Autodesk Fusion 360 part; units mm, degrees
note: some values were not read from the file. Set by a fixed rule: which sketch regions a step uses.
(part 6 of 20)
  spline S30 degree 5 poles (5.1346, -28.5878) (5.1347, -28.5879) (5.1347, -28.5881) (5.1348, -28.5884) (5.1349, -28.5889) (5.135, -28.5896) (5.1352, -28.5905) (5.1354, -28.5915) (5.1356, -28.5925) (5.1358, -28.5937) (5.1361, -28.595) (5.1363, -28.5964) (5.1367, -28.5979) (5.137, -28.5995) (5.1374, -28.6012) (5.1377, -28.603) (5.1381, -28.6049) (5.1386, -28.6069) (5.139, -28.6089) (5.1395, -28.6111) (5.14, -28.6134) (5.1406, -28.6158) (5.1411, -28.6182) (5.1417, -28.6208) (5.1423, -28.6234) (5.143, -28.6262) (5.1436, -28.629) (5.1443, -28.6319) (5.145, -28.6349) (5.1458, -28.6379) (5.1465, -28.6411) (5.1473, -28.6443) (5.1481, -28.6477) (5.149, -28.6511) (5.1499, -28.6545) (5.1508, -28.6581) (5.1517, -28.6617) (5.1527, -28.6655) (5.1536, -28.6693) (5.1546, -28.6731) (5.1557, -28.6771) (5.1567, -28.6811) (5.1578, -28.6852) (5.1589, -28.6893) (5.1601, -28.6936) (5.1613, -28.6979) (5.1625, -28.7023) (5.1637, -28.7067) (5.1649, -28.7112) (5.1662, -28.7158) (5.1675, -28.7205) (5.1689, -28.7252) (5.1702, -28.73) (5.1716, -28.7349) (5.173, -28.7398) (5.1745, -28.7448) (5.176, -28.7498) (5.1775, -28.7549) (5.179, -28.7601) (5.1806, -28.7654) (5.1822, -28.7707) (5.1838, -28.776) (5.1854, -28.7815) (5.1871, -28.7869) (5.1888, -28.7925) (5.1905, -28.7981) (5.1923, -28.8038) (5.1941, -28.8095) (5.1959, -28.8153) (5.1978, -28.8211) (5.1996, -28.827) (5.2015, -28.833) (5.2035, -28.839) (5.2054, -28.8451) (5.2074, -28.8512) (5.2094, -28.8573) (5.2115, -28.8636) (5.2136, -28.8699) (5.2157, -28.8762) (5.2178, -28.8826) (5.22, -28.889) (5.2222, -28.8955) (5.2244, -28.9021) (5.2266, -28.9087) (5.2289, -28.9153) (5.2312, -28.922) (5.2336, -28.9288) (5.2359, -28.9356) (5.2383, -28.9424) (5.2408, -28.9493) (5.2432, -28.9563) (5.2457, -28.9633) (5.2482, -28.9703) (5.2508, -28.9774) (5.2533, -28.9846) (5.2559, -28.9918) (5.2586, -28.999) (5.2612, -29.0063) (5.2639, -29.0136) (5.2666, -29.021) (5.2694, -29.0284) (5.2722, -29.0358) (5.275, -29.0433) (5.2778, -29.0509) (5.2807, -29.0585) (5.2836, -29.0661) (5.2865, -29.0738) (5.2895, -29.0815) (5.2925, -29.0893) (5.2955, -29.0971) (5.2986, -29.105) (5.3016, -29.1129) (5.3047, -29.1208) (5.3079, -29.1288) (5.3111, -29.1368) (5.3143, -29.1448) (5.3175, -29.1529) (5.3207, -29.1611) (5.324, -29.1692) (5.3273, -29.1775) (5.3307, -29.1857) (5.3341, -29.194) (5.3375, -29.2023) (5.3409, -29.2107) (5.3444, -29.2191) (5.3479, -29.2276) (5.3514, -29.2361) (5.355, -29.2446) (5.3586, -29.2531) (5.3622, -29.2617) (5.3658, -29.2704) (5.3695, -29.279) (5.3732, -29.2878) (5.377, -29.2965) (5.3807, -29.3053) (5.3846, -29.3141) (5.3884, -29.3229) (5.3922, -29.3318) (5.3961, -29.3407) (5.4001, -29.3497) (5.404, -29.3587) (5.408, -29.3677) (5.412, -29.3767) (5.4161, -29.3858) (5.4201, -29.395) (5.4242, -29.4041) (5.4284, -29.4133) (5.4325, -29.4225) (5.4367, -29.4318) (5.441, -29.441) (5.4452, -29.4504) (5.4495, -29.4597) (5.4538, -29.4691) (5.4582, -29.4785) (5.4625, -29.4879) (5.467, -29.4974) (5.4714, -29.5069) (5.4759, -29.5165) (5.4804, -29.526) (5.4849, -29.5356) (5.4895, -29.5452) (5.494, -29.5549) (5.4987, -29.5646) (5.5033, -29.5743) (5.508, -29.584) (5.5127, -29.5938) (5.5175, -29.6036) (5.5222, -29.6134) (5.527, -29.6233) (5.5319, -29.6332) (5.5367, -29.6431) (5.5416, -29.653) (5.5466, -29.663) (5.5515, -29.673) (5.5565, -29.683) (5.5615, -29.6931) (5.5666, -29.7032) (5.5717, -29.7133) (5.5768, -29.7234) (5.5819, -29.7336) (5.5871, -29.7437) (5.5923, -29.754) (5.5975, -29.7642) (5.6028, -29.7745) (5.6081, -29.7847) (5.6134, -29.7951) (5.6188, -29.8054) (5.6242, -29.8158) (5.6296, -29.8262) (5.635, -29.8366) (5.6405, -29.847) (5.646, -29.8575) (5.6515, -29.868) (5.6571, -29.8785) (5.6627, -29.889) (5.6683, -29.8996) (5.674, -29.9102) (5.6797, -29.9208) (5.6854, -29.9314) (5.6912, -29.9421) (5.697, -29.9527) (5.7028, -29.9634) (5.7086, -29.9742) (5.7145, -29.9849) (5.7204, -29.9957) (5.7263, -30.0065) (5.7323, -30.0173) (5.7383, -30.0281) (5.7443, -30.039) (5.7504, -30.0499) (5.7565, -30.0608) (5.7626, -30.0717) (5.7688, -30.0826) (5.7749, -30.0936) (5.7811, -30.1046) (5.7874, -30.1156) (5.7937, -30.1266) (5.8, -30.1377) (5.8063, -30.1487) (5.8127, -30.1598) (5.8191, -30.1709) (5.8255, -30.1821) (5.8319, -30.1932) (5.8384, -30.2044) (5.8449, -30.2156) (5.8515, -30.2268) (5.8581, -30.238) (5.8647, -30.2492) (5.8713, -30.2605) (5.878, -30.2718) (5.8847, -30.2831) (5.8914, -30.2944) (5.8982, -30.3058) (5.905, -30.3171) (5.9118, -30.3285) (5.9187, -30.3399) (5.9255, -30.3513) (5.9325, -30.3628) (5.9394, -30.3742) (5.9464, -30.3857) (5.9534, -30.3972) (5.959, -30.4064) (5.9633, -30.4133) (5.9661, -30.4179) (5.9675, -30.4202) knots 0 0 0 0 0 0 0.00416667 0.00833333 0.0125 0.01666667 0.02083333 0.025 0.02916667 0.03333333 0.0375 0.04166667 0.04583333 0.05 0.05416667 0.05833333 0.0625 0.06666667 0.07083333 0.075 0.07916667 0.08333333 0.0875 0.09166667 0.09583333 0.1 0.10416667 0.10833333 0.1125 0.11666667 0.12083333 0.125 0.12916667 0.13333333 0.1375 0.14166667 0.14583333 0.15 0.15416667 0.15833333 0.1625 0.16666667 0.17083333 0.175 0.17916667 0.18333333 0.1875 0.19166667 0.19583333 0.2 0.20416667 0.20833333 0.2125 0.21666667 0.22083333 0.225 0.22916667 0.23333333 0.2375 0.24166667 0.24583333 0.25 0.25416667 0.25833333 0.2625 0.26666667 0.27083333 0.275 0.27916667 0.28333333 0.2875 0.29166667 0.29583333 0.3 0.30416667 0.30833333 0.3125 0.31666667 0.32083333 0.325 0.32916667 0.33333333 0.3375 0.34166667 0.34583333 0.35 0.35416667 0.35833333 0.3625 0.36666667 0.37083333 0.375 0.37916667 0.38333333 0.3875 0.39166667 0.39583333 0.4 0.40416667 0.40833333 0.4125 0.41666667 0.42083333 0.425 0.42916667 0.43333333 0.4375 0.44166667 0.44583333 0.45 0.45416667 0.45833333 0.4625 0.46666667 0.47083333 0.475 0.47916667 0.48333333 0.4875 0.49166667 0.49583333 0.5 0.50416667 0.50833333 0.5125 0.51666667 0.52083333 0.525 0.52916667 0.53333333 0.5375 0.54166667 0.54583333 0.55 0.55416667 0.55833333 0.5625 0.56666667 0.57083333 0.575 0.57916667 0.58333333 0.5875 0.59166667 0.59583333 0.6 0.60416667 0.60833333 0.6125 0.61666667 0.62083333 0.625 0.62916667 0.63333333 0.6375 0.64166667 0.64583333 0.65 0.65416667 0.65833333 0.6625 0.66666667 0.67083333 0.675 0.67916667 0.68333333 0.6875 0.69166667 0.69583333 0.7 0.70416667 0.70833333 0.7125 0.71666667 0.72083333 0.725 0.72916667 0.73333333 0.7375 0.74166667 0.74583333 0.75 0.75416667 0.75833333 0.7625 0.76666667 0.77083333 0.775 0.77916667 0.78333333 0.7875 0.79166667 0.79583333 0.8 0.80416667 0.80833333 0.8125 0.81666667 0.82083333 0.825 0.82916667 0.83333333 0.8375 0.84166667 0.84583333 0.85 0.85416667 0.85833333 0.8625 0.86666667 0.87083333 0.875 0.87916667 0.88333333 0.8875 0.89166667 0.89583333 0.9 0.90416667 0.90833333 0.9125 0.91666667 0.92083333 0.925 0.92916667 0.93333333 0.9375 0.94166667 0.94583333 0.95 0.95416667 0.95833333 0.9625 0.96666667 0.97083333 0.975 0.97916667 0.98333333 0.9875 0.99166667 0.99583333 1 1 1 1 1 1
  line L63 (2.1182, -28.9671) -> (2.1183, -28.9679)
  arc A27 (6.8665, -27.918) -> (8.0125, -27.6109) centre (0, 0) ccw
  arc A28 (5.9675, -30.4202) -> (6.9214, -30.2174) centre (0, 0) ccw
  line L64 (0.9213, -29.0298) -> (0.9119, -28.7355)
  line L65 (0.9213, -29.0307) -> (0.9213, -29.0298)
  line L66 (29.0307, 0.9213) -> (29.0298, 0.9213)
  spline S31 degree 5 poles (8.0948, -27.8945) (8.0948, -27.8946) (8.0948, -27.8948) (8.0949, -27.8951) (8.0951, -27.8956) (8.0953, -27.8963) (8.0956, -27.8971) (8.0958, -27.898) (8.0962, -27.8991) (8.0965, -27.9002) (8.0969, -27.9015) (8.0973, -27.9028) (8.0978, -27.9043) (8.0983, -27.9058) (8.0988, -27.9075) (8.0994, -27.9092) (8.1, -27.9111) (8.1007, -27.913) (8.1013, -27.915) (8.102, -27.9172) (8.1028, -27.9194) (8.1036, -27.9217) (8.1044, -27.9241) (8.1052, -27.9265) (8.1061, -27.9291) (8.107, -27.9318) (8.108, -27.9345) (8.109, -27.9373) (8.11, -27.9402) (8.1111, -27.9432) (8.1121, -27.9462) (8.1133, -27.9494) (8.1144, -27.9526) (8.1156, -27.9559) (8.1169, -27.9593) (8.1181, -27.9627) (8.1194, -27.9662) (8.1208, -27.9698) (8.1222, -27.9735) (8.1236, -27.9772) (8.125, -27.9811) (8.1265, -27.9849) (8.128, -27.9889) (8.1295, -27.9929) (8.1311, -27.997) (8.1327, -28.0012) (8.1344, -28.0054) (8.1361, -28.0097) (8.1378, -28.0141) (8.1395, -28.0185) (8.1413, -28.023) (8.1432, -28.0276) (8.145, -28.0322) (8.1469, -28.0369) (8.1488, -28.0416) (8.1508, -28.0464) (8.1528, -28.0513) (8.1548, -28.0562) (8.1569, -28.0612) (8.159, -28.0663) (8.1611, -28.0714) (8.1633, -28.0765) (8.1655, -28.0818) (8.1677, -28.087) (8.17, -28.0924) (8.1723, -28.0978) (8.1747, -28.1032) (8.177, -28.1087) (8.1795, -28.1143) (8.1819, -28.1199) (8.1844, -28.1256) (8.1869, -28.1313) (8.1895, -28.1371) (8.192, -28.1429) (8.1947, -28.1488) (8.1973, -28.1547) (8.2, -28.1607) (8.2027, -28.1667) (8.2055, -28.1728) (8.2083, -28.179) (8.2111, -28.1851) (8.214, -28.1914) (8.2169, -28.1977) (8.2198, -28.204) (8.2227, -28.2104) (8.2257, -28.2168) (8.2288, -28.2233) (8.2318, -28.2298) (8.2349, -28.2363) (8.2381, -28.2429) (8.2412, -28.2496) (8.2445, -28.2563) (8.2477, -28.263) (8.251, -28.2698) (8.2543, -28.2767) (8.2576, -28.2835) (8.261, -28.2905) (8.2644, -28.2974) (8.2678, -28.3044) (8.2713, -28.3115) (8.2748, -28.3186) (8.2784, -28.3257) (8.282, -28.3329) (8.2856, -28.3401) (8.2892, -28.3473) (8.2929, -28.3546) (8.2966, -28.3619) (8.3004, -28.3693) (8.3042, -28.3767) (8.308, -28.3842) (8.3118, -28.3917) (8.3157, -28.3992) (8.3196, -28.4068) (8.3236, -28.4144) (8.3276, -28.422) (8.3316, -28.4297) (8.3357, -28.4374) (8.3398, -28.4452) (8.3439, -28.4529) (8.348, -28.4608) (8.3522, -28.4686) (8.3565, -28.4765) (8.3607, -28.4845) (8.365, -28.4924) (8.3693, -28.5004) (8.3737, -28.5085) (8.3781, -28.5165) (8.3825, -28.5246) (8.387, -28.5328) (8.3915, -28.5409) (8.396, -28.5491) (8.4006, -28.5574) (8.4052, -28.5657) (8.4098, -28.574) (8.4145, -28.5823) (8.4192, -28.5907) (8.4239, -28.5991) (8.4287, -28.6075) (8.4335, -28.616) (8.4384, -28.6244) (8.4432, -28.633) (8.4481, -28.6415) (8.4531, -28.6501) (8.458, -28.6587) (8.463, -28.6674) (8.4681, -28.676) (8.4732, -28.6847) (8.4783, -28.6935) (8.4834, -28.7022) (8.4886, -28.711) (8.4938, -28.7199) (8.499, -28.7287) (8.5043, -28.7376) (8.5096, -28.7465) (8.515, -28.7554) (8.5203, -28.7644) (8.5257, -28.7734) (8.5312, -28.7824) (8.5367, -28.7914) (8.5422, -28.8005) (8.5477, -28.8096) (8.5533, -28.8187) (8.5589, -28.8279) (8.5645, -28.837) (8.5702, -28.8462) (8.5759, -28.8555) (8.5817, -28.8647) (8.5874, -28.874) (8.5932, -28.8833) (8.5991, -28.8926) (8.605, -28.902) (8.6109, -28.9113) (8.6168, -28.9207) (8.6228, -28.9302) (8.6288, -28.9396) (8.6348, -28.9491) (8.6409, -28.9586) (8.647, -28.9681) (8.6532, -28.9776) (8.6593, -28.9872) (8.6656, -28.9968) (8.6718, -29.0064) (8.6781, -29.016) (8.6844, -29.0257) (8.6907, -29.0354) (8.6971, -29.0451) (8.7035, -29.0548) (8.7099, -29.0646) (8.7164, -29.0743) (8.7229, -29.0841) (8.7295, -29.0939) (8.736, -29.1037) (8.7426, -29.1136) (8.7493, -29.1235) (8.7559, -29.1334) (8.7626, -29.1433) (8.7694, -29.1532) (8.7762, -29.1632) (8.783, -29.1731) (8.7898, -29.1831) (8.7967, -29.1932) (8.8036, -29.2032) (8.8105, -29.2132) (8.8175, -29.2233) (8.8245, -29.2334) (8.8315, -29.2435) (8.8386, -29.2537) (8.8457, -29.2638) (8.8528, -29.274) (8.86, -29.2842) (8.8671, -29.2944) (8.8744, -29.3046) (8.8816, -29.3148) (8.8889, -29.3251) (8.8963, -29.3354) (8.9036, -29.3457) (8.911, -29.356) (8.9184, -29.3663) (8.9259, -29.3766) (8.9334, -29.387) (8.9409, -29.3974) (8.9485, -29.4078) (8.956, -29.4182) (8.9637, -29.4286) (8.9713, -29.4391) (8.979, -29.4495) (8.9867, -29.46) (8.9945, -29.4705) (9.0022, -29.481) (9.0101, -29.4915) (9.0179, -29.5021) (9.0258, -29.5127) (9.0337, -29.5232) (9.0416, -29.5338) (9.0496, -29.5444) (9.0576, -29.555) (9.0657, -29.5657) (9.0737, -29.5763) (9.0818, -29.587) (9.09, -29.5977) (9.0981, -29.6084) (9.1047, -29.6169) (9.1096, -29.6234) (9.1129, -29.6276) (9.1146, -29.6298) knots 0 0 0 0 0 0 0.00416667 0.00833333 0.0125 0.01666667 0.02083333 0.025 0.02916667 0.03333333 0.0375 0.04166667 0.04583333 0.05 0.05416667 0.05833333 0.0625 0.06666667 0.07083333 0.075 0.07916667 0.08333333 0.0875 0.09166667 0.09583333 0.1 0.10416667 0.10833333 0.1125 0.11666667 0.12083333 0.125 0.12916667 0.13333333 0.1375 0.14166667 0.14583333 0.15 0.15416667 0.15833333 0.1625 0.16666667 0.17083333 0.175 0.17916667 0.18333333 0.1875 0.19166667 0.19583333 0.2 0.20416667 0.20833333 0.2125 0.21666667 0.22083333 0.225 0.22916667 0.23333333 0.2375 0.24166667 0.24583333 0.25 0.25416667 0.25833333 0.2625 0.26666667 0.27083333 0.275 0.27916667 0.28333333 0.2875 0.29166667 0.29583333 0.3 0.30416667 0.30833333 0.3125 0.31666667 0.32083333 0.325 0.32916667 0.33333333 0.3375 0.34166667 0.34583333 0.35 0.35416667 0.35833333 0.3625 0.36666667 0.37083333 0.375 0.37916667 0.38333333 0.3875 0.39166667 0.39583333 0.4 0.40416667 0.40833333 0.4125 0.41666667 0.42083333 0.425 0.42916667 0.43333333 0.4375 0.44166667 0.44583333 0.45 0.45416667 0.45833333 0.4625 0.46666667 0.47083333 0.475 0.47916667 0.48333333 0.4875 0.49166667 0.49583333 0.5 0.50416667 0.50833333 0.5125 0.51666667 0.52083333 0.525 0.52916667 0.53333333 0.5375 0.54166667 0.54583333 0.55 0.55416667 0.55833333 0.5625 0.56666667 0.57083333 0.575 0.57916667 0.58333333 0.5875 0.59166667 0.59583333 0.6 0.60416667 0.60833333 0.6125 0.61666667 0.62083333 0.625 0.62916667 0.63333333 0.6375 0.64166667 0.64583333 0.65 0.65416667 0.65833333 0.6625 0.66666667 0.67083333 0.675 0.67916667 0.68333333 0.6875 0.69166667 0.69583333 0.7 0.70416667 0.70833333 0.7125 0.71666667 0.72083333 0.725 0.72916667 0.73333333 0.7375 0.74166667 0.74583333 0.75 0.75416667 0.75833333 0.7625 0.76666667 0.77083333 0.775 0.77916667 0.78333333 0.7875 0.79166667 0.79583333 0.8 0.80416667 0.80833333 0.8125 0.81666667 0.82083333 0.825 0.82916667 0.83333333 0.8375 0.84166667 0.84583333 0.85 0.85416667 0.85833333 0.8625 0.86666667 0.87083333 0.875 0.87916667 0.88333333 0.8875 0.89166667 0.89583333 0.9 0.90416667 0.90833333 0.9125 0.91666667 0.92083333 0.925 0.92916667 0.93333333 0.9375 0.94166667 0.94583333 0.95 0.95416667 0.95833333 0.9625 0.96666667 0.97083333 0.975 0.97916667 0.98333333 0.9875 0.99166667 0.99583333 1 1 1 1 1 1
  line L67 (-15.1575, -24.4297) -> (-15.3128, -24.6799)
  arc A29 (-16.1526, -23.7836) -> (-15.1575, -24.4297) centre (0, 0) ccw
  line L68 (2.0967, -28.6734) -> (2.1182, -28.9671)
  line L69 (24.6799, 15.3128) -> (24.4297, 15.1575)
  line L70 (3.9507, -28.7745) -> (3.9106, -28.4828)
  line L71 (6.9368, -28.2039) -> (6.8665, -27.918)
  arc A30 (0.9119, -28.7355) -> (2.0967, -28.6734) centre (0, 0) ccw
  line L72 (-16.3184, -24.0278) -> (-16.318, -24.0271)
  line L73 (-16.318, -24.0271) -> (-16.1526, -23.7836)
  arc A31 (-18.5501, -21.9649) -> (-17.6281, -22.7115) centre (0, 0) ccw
  line L74 (-15.3128, -24.6799) -> (-15.3132, -24.6806)
  arc A32 (-18.6136, -24.7898) -> (-17.8246, -25.363) centre (0, 0) ccw
  line L75 (24.6806, 15.3132) -> (24.6799, 15.3128)
  spline S32 degree 5 poles (6.9214, -30.2174) (6.9218, -30.2148) (6.9225, -30.2094) (6.9236, -30.2014) (6.925, -30.1907) (6.9267, -30.1773) (6.9284, -30.164) (6.9301, -30.1507) (6.9317, -30.1375) (6.9334, -30.1242) (6.935, -30.111) (6.9366, -30.0979) (6.9382, -30.0847) (6.9398, -30.0716) (6.9413, -30.0585) (6.9428, -30.0455) (6.9443, -30.0324) (6.9458, -30.0194) (6.9473, -30.0065) (6.9487, -29.9935) (6.9501, -29.9806) (6.9516, -29.9678) (6.9529, -29.9549) (6.9543, -29.9421) (6.9556, -29.9293) (6.957, -29.9166) (6.9583, -29.9039) (6.9596, -29.8912) (6.9608, -29.8785) (6.9621, -29.8659) (6.9633, -29.8533) (6.9645, -29.8407) (6.9657, -29.8282) (6.9669, -29.8157) (6.968, -29.8032) (6.9691, -29.7908) (6.9702, -29.7784) (6.9713, -29.766) (6.9724, -29.7537) (6.9735, -29.7414) (6.9745, -29.7291) (6.9755, -29.7169) (6.9765, -29.7047) (6.9775, -29.6925) (6.9784, -29.6803) (6.9794, -29.6682) (6.9803, -29.6562) (6.9812, -29.6441) (6.9821, -29.6321) (6.983, -29.6201) (6.9838, -29.6082) (6.9846, -29.5963) (6.9855, -29.5844) (6.9863, -29.5726) (6.987, -29.5608) (6.9878, -29.549) (6.9885, -29.5373) (6.9892, -29.5256) (6.99, -29.514) (6.9906, -29.5023) (6.9913, -29.4907) (6.992, -29.4792) (6.9926, -29.4677) (6.9932, -29.4562) (6.9938, -29.4447) (6.9944, -29.4333) (6.995, -29.422) (6.9955, -29.4106) (6.996, -29.3993) (6.9965, -29.3881) (6.997, -29.3768) (6.9975, -29.3657) (6.998, -29.3545) (6.9984, -29.3434) (6.9989, -29.3323) (6.9993, -29.3213) (6.9997, -29.3103) (7.0001, -29.2993) (7.0004, -29.2884) (7.0008, -29.2775) (7.0011, -29.2667) (7.0014, -29.2559) (7.0017, -29.2451) (7.002, -29.2344) (7.0023, -29.2237) (7.0025, -29.213) (7.0028, -29.2024) (7.003, -29.1919) (7.0032, -29.1813) (7.0034, -29.1708) (7.0035, -29.1604) (7.0037, -29.15) (7.0038, -29.1396) (7.004, -29.1293) (7.0041, -29.119) (7.0042, -29.1088) (7.0043, -29.0986) (7.0043, -29.0884) (7.0044, -29.0783) (7.0044, -29.0682) (7.0045, -29.0582) (7.0045, -29.0482) (7.0045, -29.0383) (7.0045, -29.0284) (7.0044, -29.0185) (7.0044, -29.0087) (7.0043, -28.9989) (7.0043, -28.9892) (7.0042, -28.9795) (7.0041, -28.9698) (7.004, -28.9602) (7.0038, -28.9507) (7.0037, -28.9412) (7.0036, -28.9317) (7.0034, -28.9223) (7.0032, -28.9129) (7.003, -28.9036) (7.0028, -28.8943) (7.0026, -28.8851) (7.0024, -28.8759) (7.0021, -28.8668) (7.0019, -28.8577) (7.0016, -28.8486) (7.0014, -28.8396) (7.0011, -28.8307) (7.0008, -28.8218) (7.0005, -28.8129) (7.0001, -28.8041) (6.9998, -28.7953) (6.9995, -28.7866) (6.9991, -28.778) (6.9987, -28.7694) (6.9984, -28.7608) (6.998, -28.7523) (6.9976, -28.7438) (6.9972, -28.7354) (6.9968, -28.727) (6.9963, -28.7187) (6.9959, -28.7105) (6.9954, -28.7023) (6.995, -28.6941) (6.9945, -28.686) (6.994, -28.678) (6.9936, -28.67) (6.9931, -28.662) (6.9926, -28.6541) (6.9921, -28.6463) (6.9915, -28.6385) (6.991, -28.6307) (6.9905, -28.6231) (6.9899, -28.6154) (6.9894, -28.6079) (6.9888, -28.6004) (6.9882, -28.5929) (6.9877, -28.5855) (6.9871, -28.5781) (6.9865, -28.5709) (6.9859, -28.5636) (6.9853, -28.5564) (6.9847, -28.5493) (6.9841, -28.5423) (6.9835, -28.5353) (6.9828, -28.5283) (6.9822, -28.5214) (6.9816, -28.5146) (6.9809, -28.5078) (6.9803, -28.5011) (6.9796, -28.4945) (6.9789, -28.4879) (6.9783, -28.4814) (6.9776, -28.4749) (6.9769, -28.4685) (6.9763, -28.4622) (6.9756, -28.4559) (6.9749, -28.4497) (6.9742, -28.4435) (6.9735, -28.4374) (6.9728, -28.4314) (6.9721, -28.4255) (6.9714, -28.4196) (6.9707, -28.4137) (6.97, -28.408) (6.9693, -28.4023) (6.9686, -28.3966) (6.9679, -28.3911) (6.9672, -28.3856) (6.9665, -28.3802) (6.9658, -28.3748) (6.9651, -28.3695) (6.9644, -28.3643) (6.9637, -28.3592) (6.963, -28.3541) (6.9623, -28.3491) (6.9616, -28.3442) (6.9609, -28.3393) (6.9602, -28.3345) (6.9595, -28.3298) (6.9588, -28.3252) (6.9581, -28.3206) (6.9574, -28.3161) (6.9568, -28.3117) (6.9561, -28.3074) (6.9554, -28.3031) (6.9547, -28.2989) (6.9541, -28.2948) (6.9534, -28.2908) (6.9528, -28.2868) (6.9521, -28.283) (6.9515, -28.2792) (6.9508, -28.2755) (6.9502, -28.2719) (6.9496, -28.2683) (6.949, -28.2649) (6.9484, -28.2615) (6.9478, -28.2582) (6.9472, -28.255) (6.9466, -28.2519) (6.9461, -28.2489) (6.9455, -28.246) (6.945, -28.2431) (6.9445, -28.2404) (6.9439, -28.2377) (6.9434, -28.2351) (6.9429, -28.2327) (6.9425, -28.2303) (6.942, -28.228) (6.9416, -28.2258) (6.9411, -28.2237) (6.9407, -28.2217) (6.9403, -28.2198) (6.9399, -28.218) (6.9396, -28.2163) (6.9392, -28.2147) (6.9389, -28.2132) (6.9386, -28.2118) (6.9383, -28.2106) (6.9381, -28.2094) (6.9378, -28.2083) (6.9376, -28.2074) (6.9374, -28.2065) (6.9372, -28.2058) (6.9371, -28.2053) (6.937, -28.205) (6.937, -28.2048) (6.937, -28.2047) knots -1 -1 -1 -1 -1 -1 -0.99583333 -0.99166667 -0.9875 -0.98333333 -0.97916667 -0.975 -0.97083333 -0.96666667 -0.9625 -0.95833333 -0.95416667 -0.95 -0.94583333 -0.94166667 -0.9375 -0.93333333 -0.92916667 -0.925 -0.92083333 -0.91666667 -0.9125 -0.90833333 -0.90416667 -0.9 -0.89583333 -0.89166667 -0.8875 -0.88333333 -0.87916667 -0.875 -0.87083333 -0.86666667 -0.8625 -0.85833333 -0.85416667 -0.85 -0.84583333 -0.84166667 -0.8375 -0.83333333 -0.82916667 -0.825 -0.82083333 -0.81666667 -0.8125 -0.80833333 -0.80416667 -0.8 -0.79583333 -0.79166667 -0.7875 -0.78333333 -0.77916667 -0.775 -0.77083333 -0.76666667 -0.7625 -0.75833333 -0.75416667 -0.75 -0.74583333 -0.74166667 -0.7375 -0.73333333 -0.72916667 -0.725 -0.72083333 -0.71666667 -0.7125 -0.70833333 -0.70416667 -0.7 -0.69583333 -0.69166667 -0.6875 -0.68333333 -0.67916667 -0.675 -0.67083333 -0.66666667 -0.6625 -0.65833333 -0.65416667 -0.65 -0.64583333 -0.64166667 -0.6375 -0.63333333 -0.62916667 -0.625 -0.62083333 -0.61666667 -0.6125 -0.60833333 -0.60416667 -0.6 -0.59583333 -0.59166667 -0.5875 -0.58333333 -0.57916667 -0.575 -0.57083333 -0.56666667 -0.5625 -0.55833333 -0.55416667 -0.55 -0.54583333 -0.54166667 -0.5375 -0.53333333 -0.52916667 -0.525 -0.52083333 -0.51666667 -0.5125 -0.50833333 -0.50416667 -0.5 -0.49583333 -0.49166667 -0.4875 -0.48333333 -0.47916667 -0.475 -0.47083333 -0.46666667 -0.4625 -0.45833333 -0.45416667 -0.45 -0.44583333 -0.44166667 -0.4375 -0.43333333 -0.42916667 -0.425 -0.42083333 -0.41666667 -0.4125 -0.40833333 -0.40416667 -0.4 -0.39583333 -0.39166667 -0.3875 -0.38333333 -0.37916667 -0.375 -0.37083333 -0.36666667 -0.3625 -0.35833333 -0.35416667 -0.35 -0.34583333 -0.34166667 -0.3375 -0.33333333 -0.32916667 -0.325 -0.32083333 -0.31666667 -0.3125 -0.30833333 -0.30416667 -0.3 -0.29583333 -0.29166667 -0.2875 -0.28333333 -0.27916667 -0.275 -0.27083333 -0.26666667 -0.2625 -0.25833333 -0.25416667 -0.25 -0.24583333 -0.24166667 -0.2375 -0.23333333 -0.22916667 -0.225 -0.22083333 -0.21666667 -0.2125 -0.20833333 -0.20416667 -0.2 -0.19583333 -0.19166667 -0.1875 -0.18333333 -0.17916667 -0.175 -0.17083333 -0.16666667 -0.1625 -0.15833333 -0.15416667 -0.15 -0.14583333 -0.14166667 -0.1375 -0.13333333 -0.12916667 -0.125 -0.12083333 -0.11666667 -0.1125 -0.10833333 -0.10416667 -0.1 -0.09583333 -0.09166667 -0.0875 -0.08333333 -0.07916667 -0.075 -0.07083333 -0.06666667 -0.0625 -0.05833333 -0.05416667 -0.05 -0.04583333 -0.04166667 -0.0375 -0.03333333 -0.02916667 -0.025 -0.02083333 -0.01666667 -0.0125 -0.00833333 -0.00416667 0 0 0 0 0 0
  line L76 (8.0125, -27.6109) -> (8.0945, -27.8937)
  line L77 (6.937, -28.2047) -> (6.9368, -28.2039)
  line L78 (5.0824, -28.2972) -> (5.1345, -28.587)
  arc A33 (12.1618, -28.5147) -> (13.0527, -28.1181) centre (0, 0) ccw
  arc A34 (24.4297, 15.1575) -> (23.7836, 16.1526) centre (0, 0) ccw
  line L79 (21.9649, 18.5501) -> (22.1898, 18.7401)
  arc A35 (9.7471, -27.0473) -> (10.8547, -26.6221) centre (0, 0) ccw
  arc A36 (9.1146, -29.6298) -> (10.0421, -29.3284) centre (0, 0) ccw
  line L80 (22.1898, 18.7401) -> (22.1904, 18.7406)
  line L81 (23.7836, 16.1526) -> (24.0271, 16.318)
  spline S33 degree 5 poles (10.9662, -26.8955) (10.9662, -26.8956) (10.9663, -26.8958) (10.9664, -26.8961) (10.9666, -26.8966) (10.9669, -26.8973) (10.9672, -26.8981) (10.9676, -26.899) (10.9681, -26.9) (10.9685, -26.9011) (10.9691, -26.9023) (10.9696, -26.9036) (10.9702, -26.905) (10.9709, -26.9065) (10.9716, -26.908) (10.9724, -26.9097) (10.9731, -26.9115) (10.974, -26.9134) (10.9749, -26.9153) (10.9758, -26.9173) (10.9768, -26.9195) (10.9778, -26.9217) (10.9788, -26.924) (10.9799, -26.9263) (10.9811, -26.9288) (10.9823, -26.9313) (10.9835, -26.9339) (10.9848, -26.9366) (10.9861, -26.9394) (10.9875, -26.9423) (10.9889, -26.9452) (10.9903, -26.9482) (10.9918, -26.9513) (10.9934, -26.9544) (10.9949, -26.9577) (10.9966, -26.961) (10.9982, -26.9643) (10.9999, -26.9678) (11.0017, -26.9713) (11.0035, -26.9748) (11.0053, -26.9785) (11.0072, -26.9822) (11.0091, -26.986) (11.0111, -26.9898) (11.0131, -26.9937) (11.0151, -26.9977) (11.0172, -27.0017) (11.0193, -27.0058) (11.0215, -27.01) (11.0237, -27.0142) (11.0259, -27.0185) (11.0282, -27.0228) (11.0306, -27.0272) (11.0329, -27.0317) (11.0353, -27.0362) (11.0378, -27.0408) (11.0403, -27.0454) (11.0428, -27.0501) (11.0454, -27.0549) (11.048, -27.0597) (11.0507, -27.0645) (11.0534, -27.0694) (11.0561, -27.0744) (11.0589, -27.0794) (11.0617, -27.0845) (11.0646, -27.0896) (11.0675, -27.0948) (11.0704, -27.1) (11.0734, -27.1053) (11.0764, -27.1106) (11.0795, -27.116) (11.0826, -27.1214) (11.0857, -27.1269) (11.0889, -27.1324) (11.0921, -27.138) (11.0954, -27.1436) (11.0987, -27.1493) (11.102, -27.155) (11.1054, -27.1608) (11.1088, -27.1666) (11.1123, -27.1725) (11.1158, -27.1784) (11.1193, -27.1843) (11.1229, -27.1903) (11.1265, -27.1963) (11.1301, -27.2024) (11.1338, -27.2085) (11.1376, -27.2147) (11.1413, -27.2209) (11.1451, -27.2271) (11.149, -27.2334) (11.1529, -27.2397) (11.1568, -27.2461) (11.1608, -27.2525) (11.1648, -27.259) (11.1688, -27.2654) (11.1729, -27.272) (11.177, -27.2785) (11.1812, -27.2851) (11.1854, -27.2918) (11.1896, -27.2985) (11.1939, -27.3052) (11.1982, -27.3119) (11.2025, -27.3187) (11.2069, -27.3256) (11.2113, -27.3324) (11.2158, -27.3393) (11.2203, -27.3463) (11.2248, -27.3533) (11.2294, -27.3603) (11.234, -27.3673) (11.2387, -27.3744) (11.2434, -27.3815) (11.2481, -27.3887) (11.2529, -27.3958) (11.2577, -27.4031) (11.2625, -27.4103) (11.2674, -27.4176) (11.2723, -27.4249) (11.2773, -27.4323) (11.2823, -27.4396) (11.2873, -27.447) (11.2924, -27.4545) (11.2975, -27.462) (11.3026, -27.4695) (11.3078, -27.477) (11.313, -27.4846) (11.3183, -27.4922) (11.3235, -27.4998) (11.3289, -27.5074) (11.3342, -27.5151) (11.3396, -27.5228) (11.3451, -27.5306) (11.3506, -27.5384) (11.3561, -27.5462) (11.3616, -27.554) (11.3672, -27.5618) (11.3728, -27.5697) (11.3785, -27.5776) (11.3842, -27.5856) (11.3899, -27.5936) (11.3957, -27.6015) (11.4015, -27.6096) (11.4074, -27.6176) (11.4132, -27.6257) (11.4192, -27.6338) (11.4251, -27.6419) (11.4311, -27.6501) (11.4371, -27.6582) (11.4432, -27.6665) (11.4493, -27.6747) (11.4554, -27.6829) (11.4616, -27.6912) (11.4678, -27.6995) (11.4741, -27.7078) (11.4803, -27.7162) (11.4867, -27.7246) (11.493, -27.733) (11.4994, -27.7414) (11.5058, -27.7498) (11.5123, -27.7583) (11.5188, -27.7668) (11.5253, -27.7753) (11.5319, -27.7838) (11.5385, -27.7924) (11.5452, -27.801) (11.5518, -27.8096) (11.5585, -27.8182) (11.5653, -27.8268) (11.5721, -27.8355) (11.5789, -27.8442) (11.5858, -27.8529) (11.5927, -27.8616) (11.5996, -27.8704) (11.6065, -27.8791) (11.6135, -27.8879) (11.6206, -27.8967) (11.6276, -27.9055) (11.6348, -27.9144) (11.6419, -27.9233) (11.6491, -27.9322) (11.6563, -27.9411) (11.6635, -27.95) (11.6708, -27.9589) (11.6781, -27.9679) (11.6855, -27.9769) (11.6929, -27.9859) (11.7003, -27.9949) (11.7078, -28.0039) (11.7153, -28.013) (11.7228, -28.0221) (11.7303, -28.0312) (11.7379, -28.0403) (11.7456, -28.0494) (11.7532, -28.0585) (11.7609, -28.0677) (11.7687, -28.0769) (11.7765, -28.0861) (11.7843, -28.0953) (11.7921, -28.1045) (11.8, -28.1137) (11.8079, -28.123) (11.8158, -28.1323) (11.8238, -28.1416) (11.8318, -28.1509) (11.8399, -28.1602) (11.848, -28.1695) (11.8561, -28.1789) (11.8643, -28.1882) (11.8724, -28.1976) (11.8807, -28.207) (11.8889, -28.2164) (11.8972, -28.2259) (11.9055, -28.2353) (11.9139, -28.2447) (11.9223, -28.2542) (11.9307, -28.2637) (11.9392, -28.2732) (11.9477, -28.2827) (11.9562, -28.2922) (11.9648, -28.3018) (11.9734, -28.3113) (11.982, -28.3209) (11.9907, -28.3305) (11.9994, -28.34) (12.0081, -28.3496) (12.0169, -28.3593) (12.0257, -28.3689) (12.0345, -28.3785) (12.0434, -28.3882) (12.0523, -28.3978) (12.0613, -28.4075) (12.0702, -28.4172) (12.0792, -28.4269) (12.0883, -28.4366) (12.0973, -28.4464) (12.1065, -28.4561) (12.1156, -28.4658) (12.1248, -28.4756) (12.134, -28.4854) (12.1432, -28.4951) (12.1506, -28.503) (12.1562, -28.5089) (12.16, -28.5128) (12.1618, -28.5147) knots 0 0 0 0 0 0 0.00416667 0.00833333 0.0125 0.01666667 0.02083333 0.025 0.02916667 0.03333333 0.0375 0.04166667 0.04583333 0.05 0.05416667 0.05833333 0.0625 0.06666667 0.07083333 0.075 0.07916667 0.08333333 0.0875 0.09166667 0.09583333 0.1 0.10416667 0.10833333 0.1125 0.11666667 0.12083333 0.125 0.12916667 0.13333333 0.1375 0.14166667 0.14583333 0.15 0.15416667 0.15833333 0.1625 0.16666667 0.17083333 0.175 0.17916667 0.18333333 0.1875 0.19166667 0.19583333 0.2 0.20416667 0.20833333 0.2125 0.21666667 0.22083333 0.225 0.22916667 0.23333333 0.2375 0.24166667 0.24583333 0.25 0.25416667 0.25833333 0.2625 0.26666667 0.27083333 0.275 0.27916667 0.28333333 0.2875 0.29166667 0.29583333 0.3 0.30416667 0.30833333 0.3125 0.31666667 0.32083333 0.325 0.32916667 0.33333333 0.3375 0.34166667 0.34583333 0.35 0.35416667 0.35833333 0.3625 0.36666667 0.37083333 0.375 0.37916667 0.38333333 0.3875 0.39166667 0.39583333 0.4 0.40416667 0.40833333 0.4125 0.41666667 0.42083333 0.425 0.42916667 0.43333333 0.4375 0.44166667 0.44583333 0.45 0.45416667 0.45833333 0.4625 0.46666667 0.47083333 0.475 0.47916667 0.48333333 0.4875 0.49166667 0.49583333 0.5 0.50416667 0.50833333 0.5125 0.51666667 0.52083333 0.525 0.52916667 0.53333333 0.5375 0.54166667 0.54583333 0.55 0.55416667 0.55833333 0.5625 0.56666667 0.57083333 0.575 0.57916667 0.58333333 0.5875 0.59166667 0.59583333 0.6 0.60416667 0.60833333 0.6125 0.61666667 0.62083333 0.625 0.62916667 0.63333333 0.6375 0.64166667 0.64583333 0.65 0.65416667 0.65833333 0.6625 0.66666667 0.67083333 0.675 0.67916667 0.68333333 0.6875 0.69166667 0.69583333 0.7 0.70416667 0.70833333 0.7125 0.71666667 0.72083333 0.725 0.72916667 0.73333333 0.7375 0.74166667 0.74583333 0.75 0.75416667 0.75833333 0.7625 0.76666667 0.77083333 0.775 0.77916667 0.78333333 0.7875 0.79166667 0.79583333 0.8 0.80416667 0.80833333 0.8125 0.81666667 0.82083333 0.825 0.82916667 0.83333333 0.8375 0.84166667 0.84583333 0.85 0.85416667 0.85833333 0.8625 0.86666667 0.87083333 0.875 0.87916667 0.88333333 0.8875 0.89166667 0.89583333 0.9 0.90416667 0.90833333 0.9125 0.91666667 0.92083333 0.925 0.92916667 0.93333333 0.9375 0.94166667 0.94583333 0.95 0.95416667 0.95833333 0.9625 0.96666667 0.97083333 0.975 0.97916667 0.98333333 0.9875 0.99166667 0.99583333 1 1 1 1 1 1
  line L82 (5.1345, -28.587) -> (5.1346, -28.5878)
  spline S34 degree 5 poles (13.0527, -28.1181) (13.0525, -28.1154) (13.0521, -28.11) (13.0515, -28.1019) (13.0506, -28.0911) (13.0495, -28.0777) (13.0484, -28.0644) (13.0473, -28.051) (13.0462, -28.0377) (13.0451, -28.0244) (13.0439, -28.0112) (13.0427, -27.9979) (13.0415, -27.9848) (13.0404, -27.9716) (13.0391, -27.9585) (13.0379, -27.9454) (13.0367, -27.9323) (13.0354, -27.9193) (13.0342, -27.9063) (13.0329, -27.8934) (13.0316, -27.8805) (13.0303, -27.8676) (13.029, -27.8547) (13.0276, -27.8419) (13.0263, -27.8291) (13.0249, -27.8164) (13.0236, -27.8037) (13.0222, -27.791) (13.0208, -27.7784) (13.0194, -27.7658) (13.018, -27.7532) (13.0165, -27.7406) (13.0151, -27.7281) (13.0136, -27.7157) (13.0122, -27.7032) (13.0107, -27.6908) (13.0092, -27.6785) (13.0077, -27.6661) (13.0062, -27.6539) (13.0047, -27.6416) (13.0031, -27.6294) (13.0016, -27.6172) (13, -27.605) (12.9984, -27.5929) (12.9968, -27.5809) (12.9952, -27.5688) (12.9936, -27.5568) (12.992, -27.5449) (12.9904, -27.5329) (12.9887, -27.521) (12.9871, -27.5092) (12.9854, -27.4974) (12.9838, -27.4856) (12.9821, -27.4738) (12.9804, -27.4621) (12.9787, -27.4505) (12.977, -27.4388) (12.9752, -27.4273) (12.9735, -27.4157) (12.9718, -27.4042) (12.97, -27.3927) (12.9682, -27.3813) (12.9665, -27.3699) (12.9647, -27.3585) (12.9629, -27.3472) (12.9611, -27.3359) (12.9593, -27.3247) (12.9574, -27.3135) (12.9556, -27.3023) (12.9538, -27.2912) (12.9519, -27.2801) (12.9501, -27.2691) (12.9482, -27.2581) (12.9463, -27.2471) (12.9445, -27.2362) (12.9426, -27.2253) (12.9407, -27.2145) (12.9388, -27.2037) (12.9368, -27.1929) (12.9349, -27.1822) (12.933, -27.1715) (12.9311, -27.1609) (12.9291, -27.1503) (12.9272, -27.1397) (12.9252, -27.1292) (12.9232, -27.1188) (12.9213, -27.1083) (12.9193, -27.0979) (12.9173, -27.0876) (12.9153, -27.0773) (12.9133, -27.0671) (12.9113, -27.0568) (12.9093, -27.0467) (12.9072, -27.0365) (12.9052, -27.0265) (12.9032, -27.0164) (12.9011, -27.0064) (12.8991, -26.9965) (12.8971, -26.9866) (12.895, -26.9767) (12.8929, -26.9669) (12.8909, -26.9571) (12.8888, -26.9474) (12.8867, -26.9377) (12.8847, -26.9281) (12.8826, -26.9185) (12.8805, -26.9089) (12.8784, -26.8994) (12.8763, -26.89) (12.8742, -26.8806) (12.8721, -26.8712) (12.87, -26.8619) (12.8679, -26.8526) (12.8658, -26.8434) (12.8636, -26.8342) (12.8615, -26.8251) (12.8594, -26.816) (12.8573, -26.8069) (12.8551, -26.798) (12.853, -26.789) (12.8509, -26.7801) (12.8487, -26.7713) (12.8466, -26.7625) (12.8445, -26.7537) (12.8423, -26.7451) (12.8402, -26.7364) (12.838, -26.7278) (12.8359, -26.7193) (12.8337, -26.7108) (12.8316, -26.7023) (12.8294, -26.6939) (12.8273, -26.6856) (12.8251, -26.6773) (12.823, -26.669) (12.8208, -26.6608) (12.8187, -26.6527) (12.8166, -26.6446) (12.8144, -26.6365) (12.8123, -26.6286) (12.8101, -26.6206) (12.808, -26.6127) (12.8058, -26.6049) (12.8037, -26.5971) (12.8016, -26.5894) (12.7994, -26.5817) (12.7973, -26.5741) (12.7952, -26.5665) (12.793, -26.559) (12.7909, -26.5516) (12.7888, -26.5442) (12.7867, -26.5368) (12.7845, -26.5296) (12.7824, -26.5223) (12.7803, -26.5151) (12.7782, -26.508) (12.7761, -26.5009) (12.774, -26.4939) (12.772, -26.487) (12.7699, -26.4801) (12.7678, -26.4733) (12.7657, -26.4665) (12.7637, -26.4598) (12.7616, -26.4531) (12.7596, -26.4465) (12.7575, -26.4399) (12.7555, -26.4335) (12.7534, -26.427) (12.7514, -26.4207) (12.7494, -26.4144) (12.7474, -26.4081) (12.7454, -26.4019) (12.7434, -26.3958) (12.7414, -26.3897) (12.7395, -26.3837) (12.7375, -26.3778) (12.7356, -26.3719) (12.7336, -26.3661) (12.7317, -26.3604) (12.7298, -26.3547) (12.7279, -26.3491) (12.726, -26.3435) (12.7241, -26.338) (12.7222, -26.3326) (12.7204, -26.3273) (12.7185, -26.322) (12.7167, -26.3167) (12.7149, -26.3116) (12.7131, -26.3065) (12.7113, -26.3015) (12.7095, -26.2965) (12.7077, -26.2916) (12.706, -26.2868) (12.7043, -26.282) (12.7026, -26.2774) (12.7009, -26.2728) (12.6992, -26.2682) (12.6975, -26.2638) (12.6959, -26.2594) (12.6943, -26.255) (12.6927, -26.2508) (12.6911, -26.2466) (12.6895, -26.2425) (12.688, -26.2385) (12.6864, -26.2345) (12.6849, -26.2307) (12.6834, -26.2269) (12.682, -26.2231) (12.6806, -26.2195) (12.6791, -26.2159) (12.6778, -26.2124) (12.6764, -26.209) (12.675, -26.2057) (12.6737, -26.2024) (12.6724, -26.1993) (12.6712, -26.1962) (12.6699, -26.1932) (12.6687, -26.1903) (12.6676, -26.1874) (12.6664, -26.1847) (12.6653, -26.182) (12.6642, -26.1794) (12.6631, -26.1769) (12.6621, -26.1745) (12.6611, -26.1722) (12.6602, -26.17) (12.6592, -26.1678) (12.6583, -26.1658) (12.6575, -26.1638) (12.6567, -26.1619) (12.6559, -26.1602) (12.6551, -26.1585) (12.6544, -26.1569) (12.6538, -26.1554) (12.6531, -26.154) (12.6526, -26.1527) (12.652, -26.1515) (12.6515, -26.1504) (12.651, -26.1495) (12.6506, -26.1486) (12.6503, -26.1478) (12.65, -26.1471) (12.6497, -26.1467) (12.6496, -26.1464) (12.6495, -26.1462) (12.6495, -26.1461) knots -1 -1 -1 -1 -1 -1 -0.99583333 -0.99166667 -0.9875 -0.98333333 -0.97916667 -0.975 -0.97083333 -0.96666667 -0.9625 -0.95833333 -0.95416667 -0.95 -0.94583333 -0.94166667 -0.9375 -0.93333333 -0.92916667 -0.925 -0.92083333 -0.91666667 -0.9125 -0.90833333 -0.90416667 -0.9 -0.89583333 -0.89166667 -0.8875 -0.88333333 -0.87916667 -0.875 -0.87083333 -0.86666667 -0.8625 -0.85833333 -0.85416667 -0.85 -0.84583333 -0.84166667 -0.8375 -0.83333333 -0.82916667 -0.825 -0.82083333 -0.81666667 -0.8125 -0.80833333 -0.80416667 -0.8 -0.79583333 -0.79166667 -0.7875 -0.78333333 -0.77916667 -0.775 -0.77083333 -0.76666667 -0.7625 -0.75833333 -0.75416667 -0.75 -0.74583333 -0.74166667 -0.7375 -0.73333333 -0.72916667 -0.725 -0.72083333 -0.71666667 -0.7125 -0.70833333 -0.70416667 -0.7 -0.69583333 -0.69166667 -0.6875 -0.68333333 -0.67916667 -0.675 -0.67083333 -0.66666667 -0.6625 -0.65833333 -0.65416667 -0.65 -0.64583333 -0.64166667 -0.6375 -0.63333333 -0.62916667 -0.625 -0.62083333 -0.61666667 -0.6125 -0.60833333 -0.60416667 -0.6 -0.59583333 -0.59166667 -0.5875 -0.58333333 -0.57916667 -0.575 -0.57083333 -0.56666667 -0.5625 -0.55833333 -0.55416667 -0.55 -0.54583333 -0.54166667 -0.5375 -0.53333333 -0.52916667 -0.525 -0.52083333 -0.51666667 -0.5125 -0.50833333 -0.50416667 -0.5 -0.49583333 -0.49166667 -0.4875 -0.48333333 -0.47916667 -0.475 -0.47083333 -0.46666667 -0.4625 -0.45833333 -0.45416667 -0.45 -0.44583333 -0.44166667 -0.4375 -0.43333333 -0.42916667 -0.425 -0.42083333 -0.41666667 -0.4125 -0.40833333 -0.40416667 -0.4 -0.39583333 -0.39166667 -0.3875 -0.38333333 -0.37916667 -0.375 -0.37083333 -0.36666667 -0.3625 -0.35833333 -0.35416667 -0.35 -0.34583333 -0.34166667 -0.3375 -0.33333333 -0.32916667 -0.325 -0.32083333 -0.31666667 -0.3125 -0.30833333 -0.30416667 -0.3 -0.29583333 -0.29166667 -0.2875 -0.28333333 -0.27916667 -0.275 -0.27083333 -0.26666667 -0.2625 -0.25833333 -0.25416667 -0.25 -0.24583333 -0.24166667 -0.2375 -0.23333333 -0.22916667 -0.225 -0.22083333 -0.21666667 -0.2125 -0.20833333 -0.20416667 -0.2 -0.19583333 -0.19166667 -0.1875 -0.18333333 -0.17916667 -0.175 -0.17083333 -0.16666667 -0.1625 -0.15833333 -0.15416667 -0.15 -0.14583333 -0.14166667 -0.1375 -0.13333333 -0.12916667 -0.125 -0.12083333 -0.11666667 -0.1125 -0.10833333 -0.10416667 -0.1 -0.09583333 -0.09166667 -0.0875 -0.08333333 -0.07916667 -0.075 -0.07083333 -0.06666667 -0.0625 -0.05833333 -0.05416667 -0.05 -0.04583333 -0.04166667 -0.0375 -0.03333333 -0.02916667 -0.025 -0.02083333 -0.01666667 -0.0125 -0.00833333 -0.00416667 0 0 0 0 0 0
  arc A37 (27.0873, 15.0758) -> (26.5997, 15.9204) centre (0, 0) ccw
  line L83 (12.6491, -26.1453) -> (12.5209, -25.8803)
  line L84 (12.6495, -26.1461) -> (12.6491, -26.1453)
  line L85 (22.9448, 17.8091) -> (22.9441, 17.8086)
  spline S35 degree 5 poles (-15.0758, -27.0873) (-15.0737, -27.0855) (-15.0696, -27.082) (-15.0635, -27.0767) (-15.0553, -27.0697) (-15.045, -27.061) (-15.0349, -27.0522) (-15.0247, -27.0435) (-15.0146, -27.0347) (-15.0045, -27.026) (-14.9945, -27.0173) (-14.9845, -27.0086) (-14.9745, -26.9999) (-14.9646, -26.9912) (-14.9547, -26.9825) (-14.9448, -26.9738) (-14.935, -26.9651) (-14.9252, -26.9565) (-14.9154, -26.9478) (-14.9057, -26.9392) (-14.896, -26.9305) (-14.8863, -26.9219) (-14.8767, -26.9133) (-14.8671, -26.9047) (-14.8576, -26.8961) (-14.8481, -26.8875) (-14.8386, -26.8789) (-14.8291, -26.8703) (-14.8197, -26.8618) (-14.8104, -26.8532) (-14.801, -26.8447) (-14.7917, -26.8361) (-14.7824, -26.8276) (-14.7732, -26.8191) (-14.764, -26.8106) (-14.7549, -26.8021) (-14.7457, -26.7937) (-14.7366, -26.7852) (-14.7276, -26.7767) (-14.7186, -26.7683) (-14.7096, -26.7599) (-14.7006, -26.7515) (-14.6917, -26.7431) (-14.6829, -26.7347) (-14.674, -26.7263) (-14.6652, -26.7179) (-14.6565, -26.7096) (-14.6477, -26.7012) (-14.639, -26.6929) (-14.6304, -26.6846) (-14.6218, -26.6763) (-14.6132, -26.668) (-14.6046, -26.6597) (-14.5961, -26.6514) (-14.5877, -26.6432) (-14.5792, -26.635) (-14.5708, -26.6267) (-14.5625, -26.6185) (-14.5541, -26.6103) (-14.5459, -26.6022) (-14.5376, -26.594) (-14.5294, -26.5858) (-14.5212, -26.5777) (-14.5131, -26.5696) (-14.505, -26.5615) (-14.4969, -26.5534) (-14.4889, -26.5453) (-14.4809, -26.5373) (-14.4729, -26.5292) (-14.465, -26.5212) (-14.4571, -26.5132) (-14.4493, -26.5052) (-14.4415, -26.4972) (-14.4337, -26.4893) (-14.426, -26.4813) (-14.4183, -26.4734) (-14.4106, -26.4655) (-14.403, -26.4576) (-14.3954, -26.4497) (-14.3879, -26.4419) (-14.3804, -26.434) (-14.3729, -26.4262) (-14.3655, -26.4184) (-14.3581, -26.4106) (-14.3508, -26.4029) (-14.3435, -26.3951) (-14.3362, -26.3874) (-14.3289, -26.3797) (-14.3217, -26.372) (-14.3146, -26.3643) (-14.3075, -26.3567) (-14.3004, -26.3491) (-14.2933, -26.3414) (-14.2863, -26.3339) (-14.2794, -26.3263) (-14.2724, -26.3188) (-14.2656, -26.3112) (-14.2587, -26.3037) (-14.2519, -26.2962) (-14.2451, -26.2888) (-14.2384, -26.2813) (-14.2317, -26.2739) (-14.225, -26.2665) (-14.2184, -26.2592) (-14.2119, -26.2518) (-14.2053, -26.2445) (-14.1988, -26.2372) (-14.1924, -26.2299) (-14.1859, -26.2227) (-14.1796, -26.2154) (-14.1732, -26.2082) (-14.1669, -26.201) (-14.1607, -26.1939) (-14.1544, -26.1868) (-14.1483, -26.1796) (-14.1421, -26.1726) (-14.136, -26.1655) (-14.13, -26.1585) (-14.1239, -26.1515) (-14.118, -26.1445) (-14.112, -26.1375) (-14.1061, -26.1306) (-14.1003, -26.1237) (-14.0945, -26.1168) (-14.0887, -26.11) (-14.0829, -26.1032) (-14.0772, -26.0964) (-14.0716, -26.0896) (-14.066, -26.0829) (-14.0604, -26.0762) (-14.0549, -26.0695) (-14.0494, -26.0629) (-14.0439, -26.0563) (-14.0385, -26.0497) (-14.0332, -26.0431) (-14.0278, -26.0366) (-14.0225, -26.0301) (-14.0173, -26.0236) (-14.0121, -26.0172) (-14.0069, -26.0108) (-14.0018, -26.0044) (-13.9967, -25.9981) (-13.9917, -25.9918) (-13.9867, -25.9855) (-13.9818, -25.9793) (-13.9769, -25.9731) (-13.972, -25.9669) (-13.9672, -25.9608) (-13.9624, -25.9547) (-13.9576, -25.9486) (-13.9529, -25.9426) (-13.9483, -25.9366) (-13.9437, -25.9306) (-13.9391, -25.9247) (-13.9346, -25.9188) (-13.9301, -25.913) (-13.9257, -25.9072) (-13.9213, -25.9014) (-13.9169, -25.8957) (-13.9126, -25.89) (-13.9083, -25.8843) (-13.9041, -25.8787) (-13.8999, -25.8731) (-13.8958, -25.8676) (-13.8917, -25.8621) (-13.8876, -25.8566) (-13.8836, -25.8512) (-13.8797, -25.8458) (-13.8758, -25.8405) (-13.8719, -25.8352) (-13.8681, -25.8299) (-13.8643, -25.8247) (-13.8605, -25.8195) (-13.8568, -25.8144) (-13.8532, -25.8093) (-13.8496, -25.8043) (-13.846, -25.7993) (-13.8425, -25.7944) (-13.839, -25.7895) (-13.8356, -25.7847) (-13.8322, -25.7799) (-13.8289, -25.7751) (-13.8256, -25.7704) (-13.8224, -25.7658) (-13.8192, -25.7612) (-13.816, -25.7566) (-13.8129, -25.7521) (-13.8098, -25.7476) (-13.8068, -25.7432) (-13.8039, -25.7389) (-13.8009, -25.7346) (-13.7981, -25.7304) (-13.7952, -25.7262) (-13.7925, -25.722) (-13.7897, -25.718) (-13.787, -25.7139) (-13.7844, -25.71) (-13.7818, -25.706) (-13.7793, -25.7022) (-13.7768, -25.6984) (-13.7743, -25.6947) (-13.7719, -25.691) (-13.7696, -25.6874) (-13.7673, -25.6838) (-13.765, -25.6803) (-13.7628, -25.6769) (-13.7607, -25.6735) (-13.7586, -25.6702) (-13.7565, -25.667) (-13.7545, -25.6638) (-13.7526, -25.6607) (-13.7506, -25.6577) (-13.7488, -25.6547) (-13.747, -25.6518) (-13.7452, -25.6489) (-13.7435, -25.6462) (-13.7419, -25.6435) (-13.7403, -25.6409) (-13.7387, -25.6383) (-13.7372, -25.6358) (-13.7358, -25.6334) (-13.7344, -25.6311) (-13.733, -25.6289) (-13.7317, -25.6267) (-13.7305, -25.6246) (-13.7293, -25.6226) (-13.7282, -25.6207) (-13.7271, -25.6188) (-13.7261, -25.6171) (-13.7251, -25.6154) (-13.7242, -25.6138) (-13.7233, -25.6123) (-13.7225, -25.6109) (-13.7217, -25.6096) (-13.721, -25.6083) (-13.7204, -25.6072) (-13.7198, -25.6061) (-13.7193, -25.6052) (-13.7188, -25.6043) (-13.7184, -25.6036) (-13.718, -25.6029) (-13.7178, -25.6025) (-13.7176, -25.6022) (-13.7175, -25.602) (-13.7175, -25.6019) knots -1 -1 -1 -1 -1 -1 -0.99583333 -0.99166667 -0.9875 -0.98333333 -0.97916667 -0.975 -0.97083333 -0.96666667 -0.9625 -0.95833333 -0.95416667 -0.95 -0.94583333 -0.94166667 -0.9375 -0.93333333 -0.92916667 -0.925 -0.92083333 -0.91666667 -0.9125 -0.90833333 -0.90416667 -0.9 -0.89583333 -0.89166667 -0.8875 -0.88333333 -0.87916667 -0.875 -0.87083333 -0.86666667 -0.8625 -0.85833333 -0.85416667 -0.85 -0.84583333 -0.84166667 -0.8375 -0.83333333 -0.82916667 -0.825 -0.82083333 -0.81666667 -0.8125 -0.80833333 -0.80416667 -0.8 -0.79583333 -0.79166667 -0.7875 -0.78333333 -0.77916667 -0.775 -0.77083333 -0.76666667 -0.7625 -0.75833333 -0.75416667 -0.75 -0.74583333 -0.74166667 -0.7375 -0.73333333 -0.72916667 -0.725 -0.72083333 -0.71666667 -0.7125 -0.70833333 -0.70416667 -0.7 -0.69583333 -0.69166667 -0.6875 -0.68333333 -0.67916667 -0.675 -0.67083333 -0.66666667 -0.6625 -0.65833333 -0.65416667 -0.65 -0.64583333 -0.64166667 -0.6375 -0.63333333 -0.62916667 -0.625 -0.62083333 -0.61666667 -0.6125 -0.60833333 -0.60416667 -0.6 -0.59583333 -0.59166667 -0.5875 -0.58333333 -0.57916667 -0.575 -0.57083333 -0.56666667 -0.5625 -0.55833333 -0.55416667 -0.55 -0.54583333 -0.54166667 -0.5375 -0.53333333 -0.52916667 -0.525 -0.52083333 -0.51666667 -0.5125 -0.50833333 -0.50416667 -0.5 -0.49583333 -0.49166667 -0.4875 -0.48333333 -0.47916667 -0.475 -0.47083333 -0.46666667 -0.4625 -0.45833333 -0.45416667 -0.45 -0.44583333 -0.44166667 -0.4375 -0.43333333 -0.42916667 -0.425 -0.42083333 -0.41666667 -0.4125 -0.40833333 -0.40416667 -0.4 -0.39583333 -0.39166667 -0.3875 -0.38333333 -0.37916667 -0.375 -0.37083333 -0.36666667 -0.3625 -0.35833333 -0.35416667 -0.35 -0.34583333 -0.34166667 -0.3375 -0.33333333 -0.32916667 -0.325 -0.32083333 -0.31666667 -0.3125 -0.30833333 -0.30416667 -0.3 -0.29583333 -0.29166667 -0.2875 -0.28333333 -0.27916667 -0.275 -0.27083333 -0.26666667 -0.2625 -0.25833333 -0.25416667 -0.25 -0.24583333 -0.24166667 -0.2375 -0.23333333 -0.22916667 -0.225 -0.22083333 -0.21666667 -0.2125 -0.20833333 -0.20416667 -0.2 -0.19583333 -0.19166667 -0.1875 -0.18333333 -0.17916667 -0.175 -0.17083333 -0.16666667 -0.1625 -0.15833333 -0.15416667 -0.15 -0.14583333 -0.14166667 -0.1375 -0.13333333 -0.12916667 -0.125 -0.12083333 -0.11666667 -0.1125 -0.10833333 -0.10416667 -0.1 -0.09583333 -0.09166667 -0.0875 -0.08333333 -0.07916667 -0.075 -0.07083333 -0.06666667 -0.0625 -0.05833333 -0.05416667 -0.05 -0.04583333 -0.04166667 -0.0375 -0.03333333 -0.02916667 -0.025 -0.02083333 -0.01666667 -0.0125 -0.00833333 -0.00416667 0 0 0 0 0 0
  line L86 (22.9441, 17.8086) -> (22.7115, 17.6281)
  arc A38 (25.363, 17.8246) -> (24.7898, 18.6136) centre (0, 0) ccw
  line L87 (24.0271, 16.318) -> (24.0278, 16.3184)